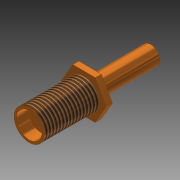
# Autodesk Inventor part: sma_female_bulkhead
Saved by Autodesk Inventor 2016 (Build 200138000, 138)
## iProperties
Created: 2013-03-02
Part Number: sma_female_bulkhead
Material: Gold
Document SubType Name: Modeling
Designer: Dave
Density: 1 g/cm^3
Appearance: Metal 1600F Hot
Author: Dave
Autodesk Inventor part; units mm, degrees
ref_plane "YZ Plane" through (0, 0, 0) normal (1, 0, 0) x (0, 1, 0)
ref_plane "XZ Plane" through (0, 0, 0) normal (0, 1, 0) x (-1, 0, 0)
ref_plane "XY Plane" through (0, 0, 0) normal (0, 0, 1) x (1, 0, 0)
sketch "Sketch1" plane through (0, 0, 0) normal (0, 0, 1) x (1, 0, 0)
  line L0 (2.3725, 4.0488) -> (4.6926, -0.0303)
  line L1 (4.6926, -0.0303) -> (2.3201, -4.0791)
  line L2 (2.3201, -4.0791) -> (-2.3725, -4.0488)
  line L3 (-2.3725, -4.0488) -> (-4.6926, 0.0303)
  line L4 (-4.6926, 0.0303) -> (-2.3201, 4.0791)
  line L5 (-2.3201, 4.0791) -> (2.3725, 4.0488)
  point P0 (0, 0)
  point P1 (0, 0)
  dimension "d0" = 8.128
  constraints: 12 end point, 1 coincident, 13 other
  measures "d0" distance between parallel lines of L2 L5
extrude "Extrusion1" add sketch "Sketch1" along normal blind 1.27
sketch "Sketch2" plane through (0, 0, 1.27) normal (0, 0, 1) x (1, 0, 0)
  circle A0 centre (0, 0) radius 3.175
  dimension "d3" = 6.35
  constraints: 1 centre point, 1 coincident
  measures "d3" diameter of A0
extrude "Extrusion2" add sketch "Sketch2" along normal blind 11.43
thread "Thread1" size "1/4-36 UNS" class "2A" standard "ANSI Unified Screw Threads" full length
sketch "Sketch3" plane through (0, 0, 12.7) normal (0, 0, 1) x (1, 0, 0)
  circle A0 centre (0, 0) radius 3.175 projected
  circle A1 centre (0, 0) radius 2.667
  dimension "d9" = 0.508
  constraints: 1 centre point
  measures "d9" radial gap between concentric circles of A0 A1
extrude "Extrusion3" cut sketch "Sketch3" against normal blind 2.54 contours A1
sketch "Sketch4" plane through (0, 0, 10.16) normal (0, 0, 1) x (1, 0, 0)
  circle A0 centre (0, 0) radius 2.667 projected
  circle A1 centre (0, 0) radius 0.4071
  constraints: 1 centre point, 1 coincident
extrude "Extrusion4" cut sketch "Sketch4" against normal blind 2.54 contours A1
sketch "Sketch5" plane through (0, 0, 0) normal (0, 0, -1) x (-1, 0, 0)
  circle A0 centre (0, 0) radius 1.905
  dimension "d14" = 3.81
  constraints: 1 centre point, 1 coincident
  measures "d14" diameter of A0
extrude "Extrusion5" add sketch "Sketch5" along normal blind 12.7
body "Solid1"
